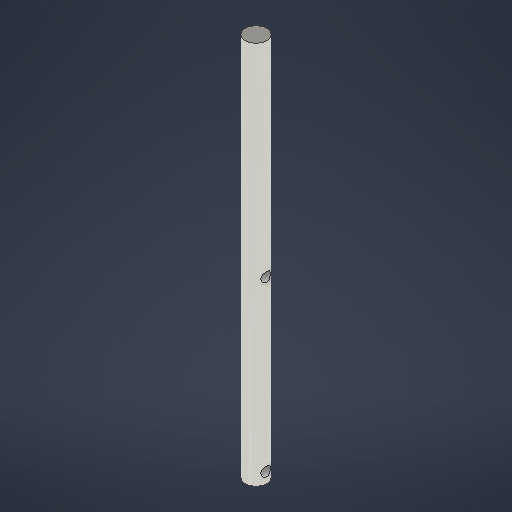
# Autodesk Inventor part: long_tibia
Saved by Autodesk Inventor 2027.1 (Build 311270010, 270A)
## iProperties
Created: 2026-08-20
Part Number: long_tibia
Material: Ogólny
Document SubType Name: Modeling
Designer: User
Density: 1 g/cm^3
Appearance: Domyślna
Author: User
Autodesk Inventor part; units mm, degrees
ref_plane "YZ Plane" through (0, 0, 0) normal (1, 0, 0) x (0, 1, 0)
ref_plane "XZ Plane" through (0, 0, 0) normal (0, 1, 0) x (-1, 0, 0)
sketch "Szkic1" plane through (0, 0, 0) normal (0, 1, 0) x (-1, 0, 0)
  circle A0 centre (0, 0) radius 5
  dimension "d0" = 10
  constraints: 1 centre point, 1 coincident
  measures "d0" diameter of A0
extrude "Wyciągnięcie proste1" add sketch "Szkic1" along normal blind 180
ref_plane "Płaszczyzna konstrukcyjna1" through (0, 90, 0) normal (0, 1, 0) x (1, 0, 0)
sketch "Szkic2" plane through (0, 90, 0) normal (0, 1, 0) x (1, 0, 0)
  circle A0 centre (0, 0) radius 18.6013
  constraints: 1 centre point, 1 coincident
sketch "Szkic3" plane through (0, 0, 0) normal (1, 0, 0) x (0, 1, 0)
  line L0 (0, 0) -> (5, 0)
  circle A0 centre (5, 0) radius 2.2
  line L1 (0, 0) -> (84, 0)
  line L2 (0, 0) -> (84, 0) construction
  circle A1 centre (84, 0) radius 2.2
  dimension "d4" = 5
  dimension "d5" = 4.4
  dimension "d6" = 84
  dimension "d7" = 0
  dimension "d8" = 4.4
  constraints: 6 end point, 3 horizontal, 2 centre point, 2 coincident, 1 collinear
  measures "d4" distance of L0.start L0.end
  measures "d5" diameter of A0
  measures "d6" distance of L0.start L1.end
  measures "d7" distance between parallel lines of L1 L2
  measures "d8" diameter of A1
extrude "Wyciągnięcie proste2" cut sketch "Szkic3" along normal mid plane 18.75
